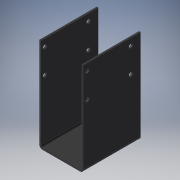
# Autodesk Inventor part: lifterMountB
Saved by Autodesk Inventor 2017 (Build 210142000, 142)
## iProperties
Created: 2017-03-09
Part Number: lifterMountB
Material: Generic
Document SubType Name: Sheet Metal
Designer: kingb
Density: 1 g/cm^3
Sheet Metal Rule: Default
Appearance: Default
Author: kingb
Autodesk Inventor part; units mm, degrees
ref_plane "YZ Plane" through (0, 0, 0) normal (1, 0, 0) x (0, 1, 0)
ref_plane "XZ Plane" through (0, 0, 0) normal (0, 1, 0) x (-1, 0, 0)
ref_plane "XY Plane" through (0, 0, 0) normal (0, 0, 1) x (1, 0, 0)
sketch "Sketch1" plane through (0, 0, 0) normal (0, 1, 0) x (-1, 0, 0)
  line L0 (0, 0) -> (42.0116, 0)
  line L1 (42.0116, 0) -> (42.0116, -59.0296)
  line L2 (42.0116, -59.0296) -> (0, -59.0296)
  line L3 (0, -59.0296) -> (0, 0)
  dimension "d0" = 42.0116
  dimension "d1" = 59.0296
  measures "d0" distance between parallel lines of L3 L1
  measures "d1" distance between parallel lines of L0 L2
extrude "Plate1" add sketch "Sketch1" along normal blind 1.5875
sketch "Sketch2" plane through (-42.0116, 1.5875, 0) normal (-1, 0, 0) x (0, -1, 0)
  line L0 (0, -59.0296) -> (0, 0)
  line L1 (0, 0) -> (-94.6023, 0)
  line L2 (-94.6023, 0) -> (-94.6023, -59.0296)
  line L3 (-94.6023, -59.0296) -> (0, -59.0296)
  constraints: 6 end point, 1 horizontal, 1 perpendicular, 1 vertical
edge flange "Flange1" height 96.1898 angle 90 thickness 1.5875 bend radius 1.5875 thickness toward (-1, 0, 0) relief straight relief width 1.5875 relief depth 0.7937 corner gap 1.5875 corner form 0 edges at (-42.0116, 1.5875, -29.5148) (0, 1.5875, -29.5148) wall of the first edge with corners at (-42.0116, 1.5875, -59.0296) (-42.0116, 1.5875, 0) (-42.0116, 96.1898, 0) (-42.0116, 96.1898, -59.0296)
bend "Bend1"
corner "Corner1"
sketch "Sketch3" plane through (1.5875, 96.1898, 0) normal (1, 0, 0) x (0, 0, -1)
  circle A0 centre (4.0046, -7.3) radius 2.0193 projected
  circle A1 centre (48.836, -7.3) radius 2.0193 projected
  circle A2 centre (48.836, -32.7) radius 2.0193 projected
  circle A3 centre (48.836, -32.7) radius 2.0193 projected
  circle A4 centre (4.0046, -32.7) radius 2.0193 projected
  point P0 (0, -96.1898)
extrude "Extrusion1" cut sketch "Sketch3" against normal up to surface (45.1866 mm away)
equation "\"d3\" = BendReliefWidth"
equation "\"d4\" = BendReliefDepth"
equation "\"d5\" = MinimumRemnant"
equation "\"d6\" = BendRadius"
equation "\"d9\" = BendRadius"
equation "\"d10\" = CornerReliefSize"
equation "\"d11\" = GapSize"
equation "\"d12\" = JacobiRadiusSize"
equation "\"BendRadius\" = Thickness"
equation "\"BendReliefWidth\" = Thickness"
equation "\"BendReliefDepth\" = 0.5 * Thickness"
equation "\"CornerReliefSize\" = 4 * Thickness"
equation "\"MinimumRemnant\" = 2 * Thickness"
equation "\"TransitionRadius\" = BendRadius"
equation "\"JacobiRadiusSize\" = Thickness"
equation "\"GapSize\" = Thickness"
equation "\"d2\" = BendRadius"
equation "\"Thickness\" = 1.5875"
body "Solid1"
